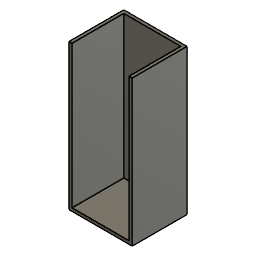
uTerreSoRo_battery_cap (Autodesk Fusion 360 design; units mm, degrees)
Autodesk Fusion 360 part; units mm, degrees
sketch "Sketch1" plane through (0, 0, 0) normal (0, 0, 1) x (1, 0, 0)
  line L0 (0, 0) -> (28, 0)
  line L1 (28, 0) -> (28, 68)
  line L2 (28, 68) -> (0, 68)
  line L3 (0, 68) -> (0, 0)
  dimension "d1" = 28
  dimension "d2" = 68
  constraint horizontal L0
  constraint vertical L1
  constraint horizontal L2
  constraint vertical L3
  constraint coincident L0.start L3.end
  measures "d1" distance of L0.start L0.end
  measures "d2" distance of L0.start L2.end
extrude "Extrude1" add sketch "Sketch1" along normal blind 25
shell "Shell1" thickness 0.5 removed faces 2 at (18.6667, 68, 8.3333) at (9.3333, 45.3333, 25)
extrude "Extrude2" add 1 faces at (9.3333, 45.3333, 0) along direction (0, 0, -1) blind 1
extrude "Extrude3" add 1 faces at (28, 45.3333, 16.3333) along direction (1, 0, 0) blind 1
extrude "Extrude4" add 1 faces at (0, 45.3333, 7.6667) along direction (-1, 0, 0) blind 1
extrude "Extrude5" add 1 faces at (9, 0, 16.3333) along direction (0, -1, 0) blind 1
